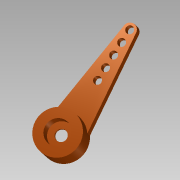
# Autodesk Inventor part: hornminiservo
Saved by Autodesk Inventor 2015 SP1 (Build 190203100, 203)
## iProperties
Created: 2015-02-03
Part Number: hornminiservo
Material: Generic
Document SubType Name: Modeling
Designer: Rafi Kurnia Putra
Density: 1 g/cm^3
Appearance: Smooth - Light Orange
Mass: 0.314786 g
Surface Area: 5.97036 cm^2
Volume: 0.314786 cm^3
Author: Rafi Kurnia Putra
Autodesk Inventor part; units mm, degrees
ref_plane "YZ Plane" through (0, 0, 0) normal (1, 0, 0) x (0, 1, 0)
ref_plane "XZ Plane" through (0, 0, 0) normal (0, 1, 0) x (-1, 0, 0)
ref_plane "XY Plane" through (0, 0, 0) normal (0, 0, 1) x (1, 0, 0)
sketch "Sketch1" plane through (0, 0, 0) normal (0, 1, 0) x (-1, 0, 0)
  circle A0 centre (0, 0) radius 4.235
  circle A1 centre (0, 0) radius 2.375
  circle A2 centre (0, 0) radius 1.11
  circle A3 centre (0, 0) radius 3.6056
  arc A4 (-1.21, -20.63) -> (1.21, -20.63) centre (0, -20.63) ccw
  line L0 (-3.38, -2.5516) -> (-1.21, -20.63)
  line L1 (3.38, -2.5516) -> (1.21, -20.63)
  circle A5 centre (0, -20.63) radius 0.75
  circle A6 centre (0, -18.18) radius 0.75
  circle A7 centre (0, -10.83) radius 0.75
  circle A8 centre (0, -13.28) radius 0.75
  circle A9 centre (0, -15.73) radius 0.75
  point P0 (0, -2.5516)
  dimension "d2" = 2.22
  dimension "d3" = 0.6294
  dimension "d14" = 1.5
  dimension "d15" = 0.46
  dimension "d16" = 1.5
  dimension "d17" = 0.95
  dimension "d18" = 1.5
  dimension "d19" = 1.5
  dimension "d20" = 1.5
  dimension "d21" = 0.95
  dimension "d22" = 0.95
  dimension "d23" = 0.95
  dimension "d26" = 4.75
  constraints: 10 centre point, 4 end point, 4 point on circle, 3 coincident, 1 vertical alignment
  measures "d2" diameter of A2
  measures "d3" radial gap between concentric circles of A0 A3
  measures "d14" diameter of A5
  measures "d15" radial gap between concentric circles of A4 A5
  measures "d16" diameter of A6
  measures "d18" diameter of A7
  measures "d19" diameter of A8
  measures "d20" diameter of A9
  measures "d26" diameter of A1
extrude "Extrusion1" add sketch "Sketch1" along normal blind 2.07 contours A0
sketch "Sketch2" plane through (0, 2.07, 0) normal (0, 1, 0) x (1, 0, 0)
  circle A0 centre (0, 0) radius 3.6056 projected
  circle A1 centre (0, 0) radius 2.375 projected
  circle A2 centre (0, 0) radius 3.6056 projected
  circle A3 centre (0, 0) radius 4.235 projected
  circle A4 centre (0, 0) radius 1.11 projected
extrude "Extrusion2" add sketch "Sketch2" along normal blind 0.63 contours A0 | A1 | A3
sketch "Sketch3" plane through (0, 2.7, 0) normal (0, 1, 0) x (1, 0, 0)
  circle A0 centre (0, 0) radius 2.375 projected
  circle A1 centre (0, 0) radius 3.6056 projected
  circle A2 centre (0, 0) radius 4.235 projected
  circle A3 centre (0, 0) radius 1.11 projected
extrude "Extrusion3" add sketch "Sketch3" along normal blind 2.81 contours A1 | A2
extrude "Extrusion4" add sketch "Sketch1" along normal blind 2.06 contours A0 L1 A4 L0
body "Solid1"
